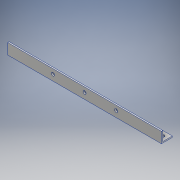
# Autodesk Inventor part: bepf_platforma_rama_bok_dlugi
Saved by Autodesk Inventor 2017 (Build 210142000, 142)
## iProperties
Created: 2016-11-24
Part Number: bepf_platforma_rama_bok_dlugi
Material: Aluminium 6061
Document SubType Name: Modeling
Designer: gagato
Density: 2.7 g/cm^3
Appearance: Aluminium — płaski
Mass: 15.1795 g
Surface Area: 82.0551 cm^2
Volume: 5.62205 cm^3
Author: gagato
Autodesk Inventor part; units mm, degrees
ref_plane "YZ Plane" through (0, 0, 0) normal (1, 0, 0) x (0, 1, 0)
ref_plane "XZ Plane" through (0, 0, 0) normal (0, 1, 0) x (-1, 0, 0)
ref_plane "XY Plane" through (0, 0, 0) normal (0, 0, 1) x (1, 0, 0)
sketch "Szkic1" plane through (0, 0, 0) normal (1, 0, 0) x (0, 1, 0)
  line L0 (0, 0) -> (12, 0)
  line L1 (12, 0) -> (12, 1.5)
  line L2 (12, 1.5) -> (1.5, 1.5)
  line L3 (1.5, 1.5) -> (1.5, 12)
  line L4 (1.5, 12) -> (0, 12)
  line L5 (0, 12) -> (0, 0)
  dimension "d0" = 12
  dimension "d1" = 1.5
  dimension "d2" = 10.5
  dimension "d3" = 10.5
  constraints: 12 end point, 5 perpendicular, 1 horizontal
  measures "d0" distance of L0.start L0.end
  measures "d1" distance of L0.end L1.end
  measures "d2" distance of L1.end L2.end
  measures "d3" distance of L2.end L3.end
extrude "Wyciągnięcie proste1" add sketch "Szkic1" along normal mid plane 170
sketch "Szkic2" plane through (-85, 0, 0) normal (0, -1, 0) x (1, 0, 0)
  line L0 (0, 12) -> (170, 12) projected
  line L1 (85, 0) -> (85, 6.75) construction
  dimension "d6" = 5.25
  constraints: 2 end point, 1 vertical
  measures "d6" distance from line of L1.end L0
hole "Otwór1" at (0, 0, 6.75) direction (0, 1, 0) diameter 3.5 end through all
sketch "Szkic3" plane through (-85, 1.5, 1.5) normal (0, 0, 1) x (1, 0, 0)
  line L0 (0, 10.5) -> (170, 10.5) construction
  line L1 (85, 10.5) -> (85, 5.25) construction
  point P0 (85, -1.5)
  dimension "d14" = 5.25
  constraints: 2 end point, 1 coincident, 1 midpoint, 1 vertical
  measures "d14" distance of L1.start L1.end
hole "Otwór2" at (0, 6.75, 1.5) direction (0, 0, -1) diameter 3.5 end through all
sketch "Szkic4" plane through (-85, 1.5, 1.5) normal (0, 0, 1) x (1, 0, 0)
  line L0 (170, 10.5) -> (170, 0) projected
  line L1 (0, 10.5) -> (170, 10.5) projected
  point P0 (85, -1.5)
  point P1 (164.75, 5.25)
  dimension "d22" = 5.25
  dimension "d23" = 5.25
  measures "d22" distance from line of L0 point (164.75, 5.25)
  measures "d23" distance from line of L1 point (164.75, 5.25)
hole "Otwór3" at (79.75, 6.75, 1.5) direction (0, 0, -1) diameter 3.5 end through all
mirror "Odbij1" about plane through (0, 0, 0) normal (1, 0, 0) of "Otwór3"
pattern_linear "Szyk prostokątny1" count 3 spacing 14.5 along (1, 0, 0) of "Otwór2" first direction both ways yes
sketch "Szkic5" plane through (-85, 1.5, 12) normal (0, 1, 0) x (1, 0, 0)
  line L0 (0, 0) -> (170, 0) construction
  circle A0 centre (85, 5.25) radius 1.75 construction
  line L1 (85, 0) -> (85, 5.25) construction
  line L2 (120, 5.25) -> (50, 5.25) construction
  point P0 (85, 12)
  dimension "d34" = 70
  constraints: 4 end point, 2 coincident, 2 midpoint, 1 horizontal, 1 vertical
  measures "d34" distance of L2.start L2.end
hole "Otwór4" at (-35, 1.5, 6.75) at (35, 1.5, 6.75) direction (0, -1, 0) diameter 3.5 end through all
